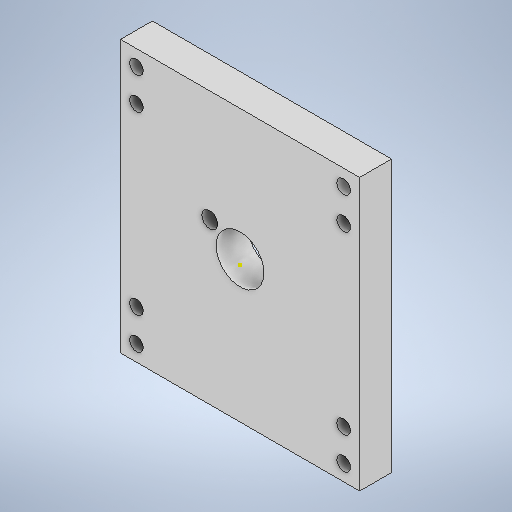
# Autodesk Inventor part: Rb PEEK - Corto con ventana
Saved by Autodesk Inventor 2025.3 (Build 293356000, 356)
## iProperties
Created: 2025-05-09
Part Number: Rb PEEK - Corto con ventana
Material: Generic
Document SubType Name: Modeling
Designer: E. Moreno
Density: 1 g/cm^3
Appearance: Default
Author: E. Moreno
Title: Rb PEEK - Corto con ventana
Autodesk Inventor part; units mm, degrees
ref_plane "YZ Plane" through (0, 0, 0) normal (1, 0, 0) x (0, 1, 0)
ref_plane "XZ Plane" through (0, 0, 0) normal (0, 1, 0) x (-1, 0, 0)
ref_plane "XY Plane" through (0, 0, 0) normal (0, 0, 1) x (1, 0, 0)
sketch "Sketch1" plane through (0, 0, 0) normal (0, 0, 1) x (1, 0, 0)
  line L0 (-37.5, -42.6) -> (37.5, -42.6)
  line L1 (37.5, -42.6) -> (37.5, 42.6)
  line L2 (37.5, 42.6) -> (-37.5, 42.6)
  line L3 (-37.5, 42.6) -> (-37.5, -42.6)
  line L4 (-37.5, -42.6) -> (37.5, 42.6) construction
  line L5 (37.5, -42.6) -> (-37.5, 42.6) construction
  point P0 (0, 0)
  dimension "d0" = 75
  dimension "d1" = 85.2
  constraints: 12 end point, 2 midpoint, 2 parallel, 1 horizontal, 1 perpendicular
  measures "d0" distance of L2.end L1.end
  measures "d1" distance of L1.end L0.end
extrude "Extrusion1" add sketch "Sketch1" along normal blind 10
sketch "Sketch4" plane through (0, 0, 10) normal (0, 0, 1) x (1, 0, 0)
  point P0 (0, 0)
sketch "Sketch5" plane through (0, 0, 10) normal (0, 0, 1) x (1, 0, 0)
  line L0 (-37.5, -42.6) -> (37.5, -42.6) projected
  line L1 (0, -42.6) -> (0, 1.6)
  circle A0 centre (0, 1.6) radius 7.5
  line L2 (0, 1.6) -> (13, 1.6)
  point P0 (0, 0)
  dimension "d21" = 44.2
  dimension "d22" = 15
  constraints: 4 end point, 1 centre point, 1 coincident, 1 horizontal, 1 midpoint, 1 vertical
  measures "d21" distance of L1.start L1.end
  measures "d22" diameter of A0
extrude "Extrusion6" cut sketch "Sketch5" against normal blind 10
sketch "Sketch6" plane through (0, 0, 10) normal (0, 0, 1) x (1, 0, 0)
  circle A0 centre (13, 6.6) radius 3.75 projected
sketch "Boceto7" plane through (0, 0, 0) normal (0, 0, -1) x (-1, 0, 0)
  circle A0 centre (0, 1.6) radius 3.9163
  circle A1 centre (0, 1.6) radius 7.5 projected
  line L0 (0, 1.6) -> (9.5, 1.6)
  line L1 (9.5, 1.6) -> (9.5, 7.6)
  circle A2 centre (9.5, 7.6) radius 2.5
  point P0 (0, 0)
  dimension "d38" = 9.5
  dimension "d39" = 6
  dimension "d40" = 5
  constraints: 4 end point, 2 centre point, 1 coincident, 1 concentric, 1 horizontal, 1 perpendicular
  measures "d38" distance of L0.start L0.end
  measures "d39" distance of L0.end L1.end
  measures "d40" diameter of A2
extrude "Extrusión7" cut sketch "Boceto7" against normal blind 10 contours A2
sketch "Boceto8" plane through (0, 0, 10) normal (0, 0, 1) x (1, 0, 0)
  circle A0 centre (-9.5, 7.6) radius 2.5 projected
sketch "Boceto9" plane through (0, 0, 0) normal (0, 0, -1) x (-1, 0, 0)
  circle A0 centre (9.5, 7.6) radius 2.5 projected
sketch "Boceto10" plane through (0, 0, 10) normal (0, 0, 1) x (1, 0, 0)
  circle A0 centre (-9.5, 7.6) radius 2.5 projected
sketch "Boceto11" plane through (0, 0, 0) normal (0, 0, -1) x (-1, 0, 0)
  circle A0 centre (9.5, 7.6) radius 2.5 projected
sketch "Sketch12" plane through (0, 0, 10) normal (0, 0, 1) x (1, 0, 0)
  point P0 (0, 0)
sketch "Sketch15" plane through (0, 0, 0) normal (0, 0, -1) x (-1, 0, 0)
  circle A0 centre (32.5, 37.6) radius 2 projected
  circle A1 centre (32.5, 37.6) radius 3.61
  line L0 (-37.5, 42.6) -> (37.5, 42.6) projected
  line L1 (0, 42.6) -> (0, 0)
  line L2 (-37.5, -42.6) -> (-37.5, 42.6) projected
  line L3 (-37.5, 0) -> (37.5, 0)
  circle A2 centre (-32.5, 37.6) radius 2
  circle A3 centre (-32.5, 37.6) radius 3.61
  circle A4 centre (32.5, -37.6) radius 2
  circle A5 centre (32.5, -37.6) radius 3.61
  circle A6 centre (-32.5, -37.6) radius 2
  circle A7 centre (-32.5, -37.6) radius 3.61
  point P0 (0, -42.6)
  dimension "d52" = 7.22
  constraints: 7 centre point, 7 symmetric about line, 4 coincident, 4 end point, 2 midpoint, 1 horizontal, 1 vertical, 6 other
  measures "d52" diameter of A1
extrude "Extrusion10" cut sketch "Sketch15" against normal blind 4.5 contours A0 | A1 | A3 | A4 | A5 | A6 | A7
sketch "Sketch13" plane through (0, 0, 10) normal (0, 0, 1) x (1, 0, 0)
  line L0 (37.5, -42.6) -> (37.5, 42.6) projected
  line L1 (37.5, -42.6) -> (32.5, -42.6)
  line L2 (-37.5, -42.6) -> (37.5, -42.6) projected
  line L3 (32.5, -42.6) -> (32.5, -37.6)
  circle A0 centre (32.5, -37.6) radius 2.15
  circle A1 centre (32.5, -37.6) radius 3.61
  line L4 (0, 0) -> (0, -42.6)
  line L5 (-37.5, 42.6) -> (-37.5, -42.6) projected
  line L6 (-37.5, 0) -> (37.5, 0)
  line L7 (-32.5, -42.6) -> (-32.5, -37.6)
  circle A2 centre (-32.5, -37.6) radius 2.15
  circle A3 centre (-32.5, -37.6) radius 3.61
  line L8 (37.5, 42.6) -> (32.5, 42.6)
  line L9 (-37.5, 42.6) -> (37.5, 42.6)
  line L10 (32.5, 42.6) -> (32.5, 37.6)
  circle A4 centre (32.5, 37.6) radius 2.15
  circle A5 centre (32.5, 37.6) radius 3.61
  line L11 (-32.5, 42.6) -> (-32.5, 37.6)
  circle A6 centre (-32.5, 37.6) radius 2.15
  circle A7 centre (-32.5, 37.6) radius 3.61
  line L12 (32.5, -37.6) -> (32.5, -27.6)
  circle A8 centre (32.5, -27.6) radius 2.15
  circle A9 centre (32.5, -27.6) radius 3.61
  line L13 (-37.5, -42.6) -> (-37.5, 42.6)
  line L14 (-37.5, -42.6) -> (-32.5, -42.6)
  line L15 (37.5, -42.6) -> (-37.5, -42.6)
  line L16 (-32.5, -42.6) -> (-32.5, -37.6)
  circle A10 centre (-32.5, -37.6) radius 2.15
  circle A11 centre (-32.5, -37.6) radius 3.61
  line L17 (-32.5, -37.6) -> (-32.5, -27.6)
  circle A12 centre (-32.5, -27.6) radius 2.15
  circle A13 centre (-32.5, -27.6) radius 3.61
  circle A14 centre (32.5, 27.6) radius 2.15
  circle A15 centre (32.5, 27.6) radius 3.61
  circle A16 centre (-32.5, 27.6) radius 2.15
  circle A17 centre (-32.5, 27.6) radius 3.61
  point P0 (0, 42.6)
  dimension "d43" = 5
  dimension "d44" = 5
  dimension "d45" = 4.3
  dimension "d46" = 7.22
  dimension "d55" = 10
  dimension "d56" = 4.3
  dimension "d57" = 7.22
  constraints: 30 end point, 27 symmetric about line, 18 centre point, 18 coincident, 3 midpoint, 3 point on line, 1 perpendicular, 1 vertical, 14 other
  measures "d43" distance of L0.start L1.end
  measures "d44" distance of L1.end L3.end
  measures "d45" diameter of A0
  measures "d46" diameter of A1
  measures "d55" distance of L12.start L12.end
  measures "d56" diameter of A8
  measures "d57" diameter of A9
extrude "Extrusion11" cut sketch "Sketch13" against normal blind 10 contours A0 L12 L3 | L3 L12 A0 | A2 L17 L7 | L7 L17 A2 | A4 | A6 | A8 | A12 | A14 | A16
sketch "Sketch16" plane through (0, 0, 0) normal (0, 0, -1) x (-1, 0, 0)
  circle A0 centre (-32.5, 27.6) radius 2.15 projected
  circle A1 centre (-32.5, 27.6) radius 3.61
  circle A2 centre (32.5, 27.6) radius 2.15 projected
  circle A3 centre (32.5, 27.6) radius 3.61
  circle A4 centre (-32.5, -27.6) radius 2.15 projected
  circle A5 centre (-32.5, -27.6) radius 3.61
  circle A6 centre (32.5, -27.6) radius 2.15 projected
  circle A7 centre (32.5, -27.6) radius 3.61
  point P0 (0, 0)
  dimension "d60" = 7.22
  dimension "d61" = 7.22
  dimension "d62" = 7.22
  dimension "d63" = 7.22
  constraints: 4 centre point, 4 coincident
  measures "d60" diameter of A1
  measures "d61" diameter of A3
  measures "d62" diameter of A5
  measures "d63" diameter of A7
extrude "Extrusion12" cut sketch "Sketch16" against normal blind 4.5
body "Solid1"
